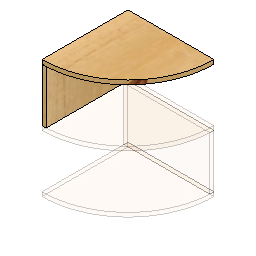
CornerShelves_B2 (Autodesk Fusion 360 design; units mm, degrees)
Autodesk Fusion 360 part; units mm, degrees
sketch "Sketch1" plane through (0, 0, 0) normal (0, 1, 0) x (1, 0, 0)
  line L0 (0, 0) -> (210, 0)
  line L1 (0, 0) -> (0, -210)
  arc A0 (0, -210) -> (210, 0) centre (0, 0) ccw
  dimension "d1" = 210
  dimension "d2" = 210
  dimension "d3" = 210
  constraint coincident L0.start L1.start
  constraint horizontal L0
  constraint perpendicular L0 L1
  measures "d1" distance of L0.start L0.end
  measures "d2" distance of L0.start L1.end
  measures "d3" radius of A0
extrude "Extrude1" add sketch "Sketch1" along normal blind 10 makes body 1
sketch "Sketch2" plane through (0, 0, 0) normal (0, 0, 1) x (1, 0, 0)
  line L0 (-10.0711, 10) -> (229.4629, 10) construction
  line L1 (0, 0) -> (0, 51.4827) construction
  line L2 (210, -0.577) -> (210, 64.8969) construction
  line L3 (210, 64.8969) -> (206.8062, 64.8969)
  line L4 (0, 10) -> (210, 10)
  line L5 (210, 10) -> (210, 140)
  line L6 (210, 140) -> (0, 140)
  line L7 (0, 140) -> (0, 10)
  dimension "d6" = 10
  dimension "d7" = 210
  dimension "d8" = 130
  dimension "d11" = 210
  constraint horizontal L0
  constraint coincident L1.start origin
  constraint perpendicular L0 L1
  constraint perpendicular L0 L2
  constraint perpendicular L2 L3
  constraint horizontal L4
  constraint vertical L5
  constraint horizontal L6
  constraint vertical L7
  constraint coincident L1 L4.start
  constraint coincident L0 L4.start
  measures "d6" distance of L1.start L0
  measures "d7" distance of L1 L2
  measures "d8" distance of L4.start L6.end
  measures "d11" distance of L5.end L6.end
extrude "Extrude2" add sketch "Sketch2" along normal blind 10 separate body makes body 2
copy_body "CopyPasteBodies1" bodies 1 makes body 3
move_body "Move1" bodies 3 to x (1, 0, 0) y (0, 1, 0) z (0, 0, 1) at (0, 140, 0)
copy_body "CopyPasteBodies2" bodies 2 makes body 4
move_body "Move2" bodies 4 to x (0, 0, 1) y (0, 1, 0) z (-1, 0, 0) at (10, 140, 0)
copy_body "CopyPasteBodies3" bodies 3 makes body 5
move_body "Move3" bodies 5 to x (1, 0, 0) y (0, 1, 0) z (0, 0, 1) at (0, 140, 0)
copy_body "CutPasteBodies1" bodies 1 2 3 removing the originals makes body 6 makes body 7 makes body 8 in component "Shelves"
copy_body "CutPasteBodies1'" bodies 4 5 removing the originals makes body 9 makes body 10 in component "Sides"
component "Shelves" placed x (1, 0, 0) y (0, 1, 0) z (0, 0, 1) at (0, 0, 0)
component "Sides" placed x (1, 0, 0) y (0, 1, 0) z (0, 0, 1) at (0, 0, 0)
named bodies: "Bottom", "RightSide", "Corner01", "Middle", "Side01", "LeftSide", "Corner (1)", "Top"
